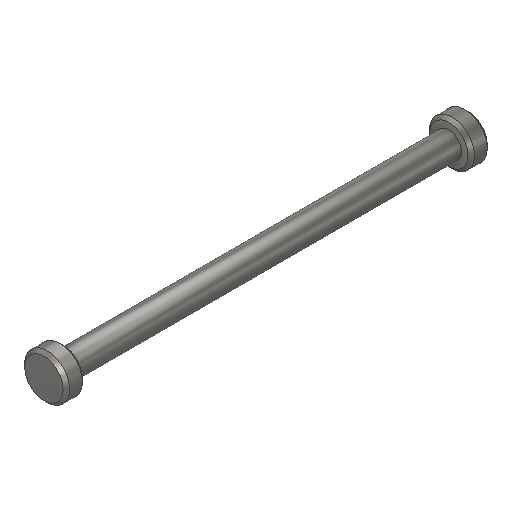
# Autodesk Inventor part: CNCT_STEEL_Outlet_door_hinge_pin
Saved by Autodesk Inventor 2025 (Build 290162010, 162A)
## iProperties
Created: 2018-09-14
Part Number: CNCT_STEEL_Outlet_door_hinge_pin
Material: Stainless Steel
Document SubType Name: Modeling
Designer: Andrzej
Density: 8 g/cm^3
Appearance: Semi-Polished
Mass: 0.974417 g
Surface Area: 2.46917 cm^2
Volume: 0.121802 cm^3
Author: Andrzej
Autodesk Inventor part; units mm, degrees
ref_plane "YZ Plane" through (0, 0, 0) normal (1, 0, 0) x (0, 1, 0)
ref_plane "XZ Plane" through (0, 0, 0) normal (0, 1, 0) x (-1, 0, 0)
ref_plane "XY Plane" through (0, 0, 0) normal (0, 0, 1) x (1, 0, 0)
sketch "Sketch1" plane through (0, 0, 0) normal (0, 0, 1) x (1, 0, 0)
  circle A0 centre (0, 0) radius 1
  circle A1 centre (0, 0) radius 1.75
  dimension "d0" = 2
  dimension "d1" = 3.5
  constraints: 2 centre point, 2 coincident
  measures "d0" diameter of A0
  measures "d1" diameter of A1
extrude "Extrusion1" add sketch "Sketch1" along normal blind 30 contours A0
extrude "Extrusion2" add sketch "Sketch1" against normal blind 1.5 contours A0 | A1
sketch "Sketch2" plane through (0, 0, 30) normal (0, 0, 1) x (1, 0, 0)
  circle A0 centre (0, 0) radius 1.75 projected
  circle A1 centre (0, 0) radius 1 projected
  circle A2 centre (0, 0) radius 1 projected
extrude "Extrusion3" add sketch "Sketch2" along normal blind 1.5 contours A0 | A1
chamfer "Chamfer1" distance 0.25 angle 45 4 edges at (-1.75, 0, 31.5) (-1.75, 0, -1.5) (-1.75, 0, 30) (-1.75, 0, 0)
body "Solid1"
